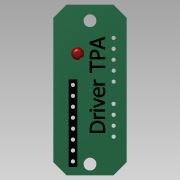
# Autodesk Inventor part: Driver TPA
Saved by Autodesk Inventor 2015 SP1 (Build 190203100, 203)
## iProperties
Created: 2015-01-28
Part Number: Driver TPA
Material: Generic
Document SubType Name: Modeling
Designer: Rafi Kurnia Putra
Density: 1 g/cm^3
Appearance: Default
Mass: 1.32746 g
Surface Area: 20.5686 cm^2
Volume: 1.32746 cm^3
Author: Rafi Kurnia Putra
Autodesk Inventor part; units mm, degrees
ref_plane "YZ Plane" through (0, 0, 0) normal (1, 0, 0) x (0, 1, 0)
ref_plane "XZ Plane" through (0, 0, 0) normal (0, 1, 0) x (-1, 0, 0)
ref_plane "XY Plane" through (0, 0, 0) normal (0, 0, 1) x (1, 0, 0)
sketch "Sketch1" plane through (0, 0, 0) normal (0, 1, 0) x (-1, 0, 0)
  line L0 (5.5, 19.825) -> (-5.5, 19.825)
  line L1 (-8.5, 16.825) -> (-8.5, -16.825)
  line L2 (-5.5, -19.825) -> (5.5, -19.825)
  line L3 (8.5, -16.825) -> (8.5, 16.825)
  line L4 (8.5, 19.825) -> (-8.5, -19.825) construction
  line L5 (-8.5, 19.825) -> (8.5, -19.825) construction
  line L6 (-5.5, 19.825) -> (-8.5, 16.825)
  line L7 (5.5, 19.825) -> (8.5, 16.825)
  line L8 (8.5, -16.825) -> (5.5, -19.825)
  line L9 (-5.5, -19.825) -> (-8.5, -16.825)
  circle A0 centre (3.9654, 16.6011) radius 0.5
  circle A1 centre (3.9654, 14.0611) radius 0.5
  circle A2 centre (3.9654, 11.5211) radius 0.5
  circle A3 centre (3.9654, 6.4411) radius 0.5
  circle A4 centre (3.9654, 3.9011) radius 0.5
  circle A5 centre (3.9654, 1.3611) radius 0.5
  circle A6 centre (3.9654, -1.1789) radius 0.5
  line L10 (4.9485, 17.9314) -> (2.9084, 17.9314)
  line L11 (2.9084, 17.9314) -> (2.9084, -2.5092)
  line L12 (2.9084, -2.5092) -> (4.9485, -2.5092)
  line L13 (4.9485, -2.5092) -> (4.9485, 17.9314)
  circle A7 centre (2.8556, -8.4694) radius 1.5
  circle A8 centre (-5.4926, 10.8475) radius 0.5
  circle A9 centre (-5.4926, 8.3075) radius 0.5
  circle A10 centre (-5.4926, 5.7675) radius 0.5
  circle A11 centre (-5.4926, 3.2275) radius 0.5
  circle A12 centre (-5.4926, -1.9498) radius 0.5
  circle A13 centre (-5.4926, -4.4898) radius 0.5
  circle A14 centre (-5.4926, -7.0298) radius 0.5
  circle A15 centre (-5.4926, -9.5698) radius 0.5
  circle A16 centre (-5.5, -12.1098) radius 0.5
  circle A17 centre (0, -16.105) radius 1.5
  circle A18 centre (0, 17.225) radius 1.5
  circle A19 centre (3.9285, 8.9811) radius 0.5
  point P0 (0, 0)
  dimension "d0" = 17
  dimension "d1" = 39.65
  dimension "d2" = 3
  dimension "d3" = 3
  dimension "d4" = 3
  dimension "d5" = 3
  dimension "d6" = 3
  dimension "d7" = 3
  dimension "d8" = 3
  dimension "d9" = 3
  dimension "d10" = 1
  dimension "d11" = 1
  dimension "d12" = 1
  dimension "d13" = 1
  dimension "d14" = 1
  dimension "d15" = 1
  dimension "d16" = 1
  dimension "d17" = 2.54
  dimension "d18" = 2.54
  dimension "d19" = 2.54
  dimension "d20" = 2.54
  dimension "d21" = 2.54
  dimension "d23" = 3
  dimension "d24" = 1
  dimension "d25" = 1
  dimension "d26" = 1
  dimension "d27" = 1
  dimension "d28" = 2.54
  dimension "d29" = 2.54
  dimension "d30" = 2.54
  dimension "d31" = 1
  dimension "d32" = 1
  dimension "d33" = 1
  dimension "d34" = 1
  dimension "d35" = 2.54
  dimension "d36" = 2.54
  dimension "d37" = 2.54
  dimension "d39" = 2.54
  dimension "d51" = 3
  dimension "d52" = 3
  dimension "d53" = 2.6
  dimension "d54" = 3.72
  dimension "d59" = 33.33
  dimension "d60" = 1
  dimension "d61" = 2.54
  dimension "d62" = 2.54
  dimension "d63" = 1.3303
  dimension "d64" = 1.3303
  constraints: 28 end point, 20 centre point, 8 point on line, 8 vertical alignment, 4 parallel, 2 horizontal, 2 midpoint, 2 perpendicular
  measures "d0" distance of L5.end L4.end
  measures "d1" distance of L4.end L5.start
  measures "d2" distance of L0.end L5.start
  measures "d3" distance of L1.start L5.start
  measures "d4" distance of L0.start L4.start
  measures "d5" distance of L3.end L4.start
  measures "d6" distance of L3.start L5.end
  measures "d7" distance of L2.end L5.end
  measures "d8" distance of L2.start L4.end
  measures "d9" distance of L1.end L4.end
  measures "d10" diameter of A0
  measures "d11" diameter of A1
  measures "d12" diameter of A2
  measures "d13" diameter of A3
  measures "d14" diameter of A4
  measures "d15" diameter of A5
  measures "d16" diameter of A6
  measures "d17" distance of A1.centre A0.centre
  measures "d18" distance of A1.centre A2.centre
  measures "d19" distance of A4.centre A3.centre
  measures "d20" distance of A4.centre A5.centre
  measures "d21" distance of A5.centre A6.centre
  measures "d23" diameter of A7
  measures "d24" diameter of A8
  measures "d25" diameter of A9
  measures "d26" diameter of A10
  measures "d27" diameter of A11
  measures "d28" distance of A9.centre A8.centre
  measures "d29" distance of A9.centre A10.centre
  measures "d30" distance of A10.centre A11.centre
  measures "d31" diameter of A12
  measures "d32" diameter of A13
  measures "d33" diameter of A14
  measures "d34" diameter of A15
  measures "d35" distance of A13.centre A12.centre
  measures "d36" distance of A13.centre A14.centre
  measures "d37" distance of A14.centre A15.centre
  measures "d39" distance of A16.centre A15.centre
  measures "d51" diameter of A17
  measures "d52" diameter of A18
  measures "d53" distance from line of L0 A18.centre
  measures "d54" distance from line of A17.centre L2
  measures "d59" distance of A18.centre A17.centre
  measures "d60" diameter of A19
  measures "d61" vertical distance of A19.centre A3.centre
  measures "d62" vertical distance of A19.centre A2.centre
  measures "d63" distance from line of A6.centre L12
  measures "d64" distance from line of L10 A0.centre
extrude "Extrusion2" add sketch "Sketch1" along normal blind 8.4 contours L13 L12 L11 L10 | A19
extrude "Extrusion3" add sketch "Sketch1" along normal blind 5 contours A7
extrude "Extrusion4" cut sketch "Sketch1" along normal blind 1.7 contours L7 L3 L8 L2 L9 L1 L6 L0 | A17 | A18
extrude "Extrusion5" add sketch "Sketch1" along normal blind 1.7 contours L7 L3 L8 L2 L9 L1 L6 L0 | A17 | A18
fillet "Fillet1" radius 1 1 edges at (-1.3556, 5, -8.4694)
sketch "Sketch2" plane through (0, 1.7, 0) normal (0, 1, 0) x (1, 0, 0)
  line L0 (-0.041, -10.2921) -> (-0.041, 12.3756) construction
  line L1 (-0.041, 12.3756) -> (3.5412, 12.3756) construction
  line L2 (3.5412, 12.3756) -> (3.5412, -10.2921) construction
  line L3 (3.5412, -10.2921) -> (-0.041, -10.2921) construction
  point P0 (0, 0)
  constraints: 2 other
extrude "Extrusion6" cut sketch "Sketch1" against normal blind 10 contours A17 | A18
extrude "Extrusion7" cut sketch "Sketch1" along normal through all contours A17 | A18
extrude "Extrusion8" cut sketch "Sketch1" along normal up to next contours A19
equation "\"d3\" = d2"
equation "\"d4\" = d2"
equation "\"d5\" = d4"
equation "\"d6\" = d2"
equation "\"d7\" = d6"
equation "\"d8\" = d2"
equation "\"d9\" = d8"
body "Solid1"
